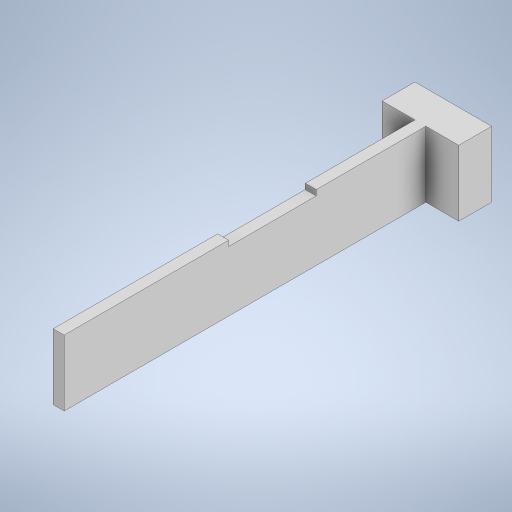
# Autodesk Inventor part: light_divider
Saved by Autodesk Inventor 2024 (Build 280153000, 153)
## iProperties
Created: 2024-05-17
Part Number: light_divider
Material: Generic
Document SubType Name: Modeling
Designer: david
Density: 1 g/cm^3
Appearance: Default
Author: david
Autodesk Inventor part; units mm, degrees
ref_plane "YZ Plane" through (0, 0, 0) normal (1, 0, 0) x (0, 1, 0)
ref_plane "XZ Plane" through (0, 0, 0) normal (0, 1, 0) x (-1, 0, 0)
ref_plane "XY Plane" through (0, 0, 0) normal (0, 0, 1) x (1, 0, 0)
sketch "Sketch1" plane through (0, 0, 0) normal (0, 1, 0) x (-1, 0, 0)
  line L0 (0, 0) -> (0, -33)
  line L1 (0, 0) -> (1, 0)
  line L2 (1, 0) -> (1, -33)
  line L3 (1, -33) -> (4, -33)
  line L4 (4, -33) -> (4, -36)
  line L5 (4, -36) -> (-3, -36)
  line L6 (-3, -36) -> (-3, -33)
  line L7 (-3, -33) -> (0, -33)
  dimension "d0" = 33
  dimension "d1" = 1
  dimension "d2" = 33
  dimension "d3" = 3
  dimension "d4" = 3
  dimension "d5" = 7
  constraints: 16 end point, 4 perpendicular, 2 horizontal, 1 point on line, 1 vertical
  measures "d0" distance of L0.start L0.end
  measures "d1" distance of L0.start L1.end
  measures "d2" distance of L1.end L2.end
  measures "d3" distance of L2.end L3.end
  measures "d4" distance of L3.end L4.end
  measures "d5" distance of L4.end L5.end
extrude "Extrusion1" add sketch "Sketch1" along normal blind 6
sketch "Sketch2" plane through (0, 6, 0) normal (0, 1, 0) x (1, 0, 0)
  line L0 (-1, 33) -> (-1, 0) projected
  line L1 (-1, 0) -> (-1, 15)
  line L2 (-1, 0) -> (-1, 23)
  line L3 (-1, 15) -> (0, 15)
  line L4 (0, 0) -> (0, 33) projected
  line L5 (-1, 23) -> (0, 23)
  line L6 (0, 15) -> (0, 23)
  dimension "d8" = 15
  dimension "d9" = 23
  constraints: 10 end point, 4 point on line, 1 horizontal, 1 parallel, 1 perpendicular
  measures "d8" distance of L0.end L1.end
  measures "d9" distance of L0.end L2.end
extrude "Extrusion2" cut sketch "Sketch2" against normal blind 0.5
body "Solid1"
